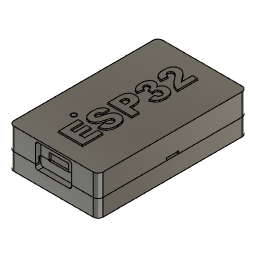
ESP32 BOX YT v12 (Autodesk Fusion 360 design; units mm, degrees)
Autodesk Fusion 360 part; units mm, degrees
(part 1 of 2)
sketch "Sketch1" plane through (0, 0, 0) normal (0, 0, 1) x (1, 0, 0) in component "Board"
  line L0 (13.95, 0) -> (-13.95, 0)
  line L1 (-13.95, 0) -> (-13.95, 54.4)
  line L2 (-13.95, 54.4) -> (13.95, 54.4)
  line L3 (13.95, 54.4) -> (13.95, 0)
  line L4 (13.95, 0) -> (-13.95, 54.4) construction
  line L5 (-13.95, 0) -> (13.95, 54.4) construction
  line L6 (0, 1.75) -> (0, 22.5)
  line L7 (1.75, 0) -> (22.5, 0)
  line L8 (9, 54.4) -> (-9, 54.4)
  line L9 (-9, 54.4) -> (-9, 28.9)
  line L10 (-9, 28.9) -> (9, 28.9)
  line L11 (9, 28.9) -> (9, 54.4)
  line L12 (9, 54.4) -> (-9, 28.9) construction
  line L13 (-9, 54.4) -> (9, 28.9) construction
  line L14 (3.9, 5.7) -> (-3.9, 5.7)
  line L15 (-3.9, 5.7) -> (-3.9, -1)
  line L16 (-3.9, -1) -> (3.9, -1)
  line L17 (3.9, -1) -> (3.9, 5.7)
  line L18 (3.9, 5.7) -> (-3.9, -1) construction
  line L19 (-3.9, 5.7) -> (3.9, -1) construction
  line L20 (-7.6, 13.8) -> (-8.4, 13.8)
  line L21 (-8.4, 13.8) -> (-8.4, 12.2)
  line L22 (-8.4, 12.2) -> (-7.6, 12.2)
  line L23 (-7.6, 12.2) -> (-7.6, 13.8)
  line L24 (-7.6, 13.8) -> (-8.4, 12.2) construction
  line L25 (-8.4, 13.8) -> (-7.6, 12.2) construction
  point P0 (0, 27.2)
  point P1 (0, 41.65)
  point P2 (0, 2.35)
  point P3 (-8, 13)
  dimension "d3" = 27.9
  dimension "d4" = 54.4
  dimension "d5" = 18
  dimension "d6" = 25.5
  dimension "d7" = 7.8
  dimension "d8" = 6.7
  dimension "d9" = 1
  dimension "d10" = 0.8
  dimension "d11" = 1.6
  dimension "d12" = 8
  dimension "d13" = 13
  constraint horizontal L0
  constraint perpendicular L0 L1
  constraint parallel L0 L2
  constraint parallel L1 L3
  constraint coincident L4 P0
  constraint coincident L5 P0
  constraint coincident P0 L6
  constraint collinear L0 L7
  constraint horizontal L8
  constraint perpendicular L8 L9
  constraint parallel L8 L10
  constraint parallel L9 L11
  constraint coincident L12 P1
  constraint coincident L13 P1
  constraint coincident L6 P1
  constraint collinear L2 L8
  constraint horizontal L14
  constraint perpendicular L14 L15
  constraint parallel L14 L16
  constraint parallel L15 L17
  constraint coincident L18 P2
  constraint coincident L19 P2
  constraint coincident L6 P2
  constraint horizontal L20
  constraint perpendicular L20 L21
  constraint parallel L20 L22
  constraint parallel L21 L23
  constraint coincident L24 P3
  constraint coincident L25 P3
  measures "d3" distance of L1.end L2.end
  measures "d4" distance of L0.end L1.end
  measures "d5" distance of L9.end L10.end
  measures "d6" distance of L8.end L9.end
  measures "d7" distance of L15.end L16.end
  measures "d8" distance of L14.end L15.end
  measures "d9" distance of L0 L16
  measures "d10" distance of L21.end L22.end
  measures "d11" distance of L20.end L21.end
  measures "d12" horizontal distance of origin P3
  measures "d13" vertical distance of origin P3
extrude "Extrude1" add sketch "Sketch1" against normal blind 1.6 contours L0 L1 L2 L3 L7 L9 L10 L11 L14 L15 L17 | L0 L7 L14 L15 L17 | L2 L8 L9 L10 L11 | L20 L21 L22 L23 makes body 1 in component "Board"
extrude "Extrude2" add sketch "Sketch1" along normal blind 3.4 contours L2 L8 L9 L10 L11 bodies 1 in component "Board"
extrude "Extrude3" add sketch "Sketch1" along normal blind 0.7 contours L20 L21 L22 L23 bodies 1 in component "Board"
extrude "Extrude4" add sketch "Sketch1" along normal blind 2.7 contours L0 L7 L15 L16 L17 | L0 L7 L14 L15 L17 bodies 1 in component "Board"
extrude "Extrude5" add sketch "Sketch1" against normal blind 0.2 contours L0 L7 L15 L16 L17 bodies 1 in component "Board"
sketch "Sketch1 (2)" plane through (0, 0, 0) normal (0, 0, 1) x (1, 0, 0)
  line L0 (14.25, -0.3) -> (-14.25, -0.3)
  line L1 (-14.25, -0.3) -> (-14.25, 54.7)
  line L2 (-14.25, 54.7) -> (14.25, 54.7)
  line L3 (14.25, 54.7) -> (14.25, -0.3)
  line L4 (14.25, -0.3) -> (-14.25, 54.7) construction
  line L5 (-14.25, -0.3) -> (14.25, 54.7) construction
  line L6 (0, 1.75) -> (0, 22.5)
  line L7 (-17.25, -3.3) -> (-17.25, 57.7)
  line L8 (-17.25, 57.7) -> (17.25, 57.7)
  line L9 (17.25, 57.7) -> (17.25, -3.3)
  line L10 (17.25, -3.3) -> (-17.25, -3.3)
  line L11 (-15.65, -1.7) -> (-15.65, 56.1)
  line L12 (-15.65, 56.1) -> (15.65, 56.1)
  line L13 (15.65, 56.1) -> (15.65, -1.7)
  line L14 (15.65, -1.7) -> (-15.65, -1.7)
  line L15 (-15.85, -1.9) -> (-15.85, 56.3)
  line L16 (-15.85, 56.3) -> (15.85, 56.3)
  line L17 (15.85, 56.3) -> (15.85, -1.9)
  line L18 (15.85, -1.9) -> (-15.85, -1.9)
  line L19 (16.55, 17.4) -> (14.95, 17.4)
  line L20 (14.95, 17.4) -> (14.95, 9.8)
  line L21 (14.95, 9.8) -> (16.55, 9.8)
  line L22 (16.55, 9.8) -> (16.55, 17.4)
  line L23 (16.55, 17.4) -> (14.95, 9.8) construction
  line L24 (14.95, 17.4) -> (16.55, 9.8) construction
  point P0 (0, 27.2)
  point P1 (15.75, 13.6)
  point P2 (15.75, 13.6)
  dimension "d32" = 28.5
  dimension "d33" = 55
  dimension "d34" = 0.3
  dimension "d71" = -1.4
  dimension "d72" = -1.6
  dimension "d100" = 13.6
  dimension "d101" = 15.75
  dimension "d107" = 1.6
  dimension "d108" = 7.6
  constraint horizontal L0
  constraint perpendicular L0 L1
  constraint parallel L0 L2
  constraint parallel L1 L3
  constraint coincident L4 P0
  constraint coincident L5 P0
  constraint coincident P0 L6
  constraint horizontal L19
  constraint perpendicular L19 L20
  constraint parallel L19 L21
  constraint parallel L20 L22
  constraint coincident L23 P2
  constraint coincident L24 P2
  constraint coincident P2 P1
  measures "d32" distance of L1.end L2.end
  measures "d33" distance of L0.end L1.end
  measures "d34" distance of origin L0
  measures "d100" vertical distance of origin P2
  measures "d101" horizontal distance of origin P2
  measures "d107" distance of L20.end L21.end
  measures "d108" distance of L19.end L20.end
extrude "Extrude1'" add sketch "Sketch1 (2)" against normal blind 9 separate body contours L0 L1 L2 L3 | L7 L8 L9 L10 | L11 L12 L13 L14 L15 L16 L17 L18 L19 L21 | L11 L12 L13 L14 L19 L20 L21 | L13 L19 L20 L21 | L13 L17 L19 L21 | L17 L19 L21 L22 makes body 2 in component "Bottom"
extrude "Extrude2'" cut sketch "Sketch1 (2)" against normal blind 8 contours L0 L1 L2 L3 bodies 2 in component "Bottom"
extrude "Extrude1''" add sketch "Sketch1 (2)" along normal blind 7 separate body contours L0 L1 L2 L3 | L7 L8 L9 L10 | L11 L12 L13 L14 L15 L16 L17 L18 L19 L21 | L11 L12 L13 L14 L19 L20 L21 | L13 L19 L20 L21 | L13 L17 L19 L21 | L17 L19 L21 L22 makes body 3 in component "Top"
extrude "Extrude2''" cut sketch "Sketch1 (2)" along normal blind 6 contours L0 L1 L2 L3 bodies 3 in component "Top"
sketch "Sketch1 (3)" plane through (0, 0, -9) normal (0, 0, -1) x (1, 0, 0) in component "Bottom"
  line L0 (17.25, -57.7) -> (17.25, 3.3)
  line L1 (17.25, 3.3) -> (-17.25, 3.3)
  line L2 (-17.25, 3.3) -> (-17.25, -57.7)
  line L3 (-17.25, -57.7) -> (17.25, -57.7)
  line L4 (7.5, -42.2) -> (-7.5, -42.2)
  line L5 (-7.5, -42.2) -> (-7.5, -12.2)
  line L6 (-7.5, -12.2) -> (7.5, -12.2)
  line L7 (7.5, -12.2) -> (7.5, -42.2)
  line L8 (7.5, -42.2) -> (-7.5, -12.2) construction
  line L9 (-7.5, -42.2) -> (7.5, -12.2) construction
  line L10 (0, -1.75) -> (0, -22.5)
  line L11 (16.55, -17.4) -> (14.95, -17.4)
  line L12 (14.95, -17.4) -> (14.95, -9.8)
  line L13 (14.95, -9.8) -> (16.55, -9.8)
  line L14 (16.55, -9.8) -> (16.55, -17.4)
  line L15 (16.55, -17.4) -> (14.95, -9.8) construction
  line L16 (14.95, -17.4) -> (16.55, -9.8) construction
  line L17 (16.55, -19.6) -> (14.95, -19.6)
  line L18 (14.95, -19.6) -> (14.95, -7.6)
  line L19 (14.95, -7.6) -> (16.55, -7.6)
  line L20 (16.55, -7.6) -> (16.55, -19.6)
  line L21 (16.55, -19.6) -> (14.95, -7.6) construction
  line L22 (14.95, -19.6) -> (16.55, -7.6) construction
  point P0 (0, -27.2)
  point P1 (15.75, -13.6)
  point P2 (15.75, -13.6)
  dimension "d56" = 15
  dimension "d57" = 30
  dimension "d58" = 27.2
  dimension "d123" = 1.6
  dimension "d124" = 7.6
  dimension "d125" = 1.6
  dimension "d126" = 12
  dimension "d127" = 15.75
  dimension "d128" = 13.6
  constraint horizontal L4
  constraint perpendicular L4 L5
  constraint parallel L4 L6
  constraint parallel L5 L7
  constraint coincident L8 P0
  constraint coincident L9 P0
  constraint coincident P0 L10
  constraint horizontal L11
  constraint perpendicular L11 L12
  constraint parallel L11 L13
  constraint parallel L12 L14
  constraint coincident L15 P2
  constraint coincident L16 P2
  constraint horizontal L17
  constraint perpendicular L17 L18
  constraint parallel L17 L19
  constraint parallel L18 L20
  constraint coincident L21 P2
  constraint coincident L22 P2
  constraint coincident P2 P1
  measures "d56" distance of L5.end L6.end
  measures "d57" distance of L4.end L5.end
  measures "d58" distance of origin P0
  measures "d123" distance of L12.end L13.end
  measures "d124" distance of L11.end L12.end
  measures "d125" distance of L18.end L19.end
  measures "d126" distance of L17.end L18.end
  measures "d127" horizontal distance of origin P2
  measures "d128" vertical distance of origin P2
extrude "Extrude5'" add sketch "Sketch1 (3)" against normal blind 7.3 contours L4 L5 L6 L7 bodies 2 in component "Bottom"
sketch "Sketch1 (4)" plane through (0, 0, 7) normal (0, 0, 1) x (-1, 0, 0) in component "Top"
  line L0 (-17.25, 3.3) -> (-17.25, -57.7)
  line L1 (-17.25, -57.7) -> (17.25, -57.7)
  line L2 (17.25, -57.7) -> (17.25, 3.3)
  line L3 (17.25, 3.3) -> (-17.25, 3.3)
  line L4 (-5, -34.4) -> (5, -34.4)
  line L5 (5, -34.4) -> (5, -44.4)
  line L6 (5, -44.4) -> (-5, -44.4)
  line L7 (-5, -44.4) -> (-5, -34.4)
  line L8 (-5, -34.4) -> (5, -44.4) construction
  line L9 (5, -34.4) -> (-5, -44.4) construction
  line L10 (-2.5, -0.5) -> (2.5, -0.5)
  line L11 (2.5, -0.5) -> (2.5, -5.5)
  line L12 (2.5, -5.5) -> (-2.5, -5.5)
  line L13 (-2.5, -5.5) -> (-2.5, -0.5)
  line L14 (-2.5, -0.5) -> (2.5, -5.5) construction
  line L15 (2.5, -0.5) -> (-2.5, -5.5) construction
  line L16 (0, -1.75) -> (0, -22.5)
  circle A0 centre (8, -13) radius 1.075
  circle A1 centre (8, -13) radius 3.075
  line L17 (-13.95, 0) -> (-13.95, -54.4) construction
  line L18 (-13.95, -54.4) -> (13.95, -54.4) construction
  line L19 (13.95, -54.4) -> (13.95, 0) construction
  line L20 (13.95, 0) -> (-13.95, 0) construction
  point P0 (0, -39.4)
  point P1 (0, -3)
  point P2 (8, -13)
  dimension "d61" = 10
  dimension "d62" = 10
  dimension "d63" = 5
  dimension "d64" = 5
  dimension "d65" = 3
  dimension "d66" = 39.4
  dimension "d143" = 2.15
  dimension "d144" = 2
  dimension "d162" = 10
  dimension "d163" = 54.4
  dimension "d164" = 27.9
  text T0 "ESP32" font "Arial Black" height 10 align centre middle in box 54.4 x 27.9 at (-13.95, 0) x (0, -1) y (1, 0) spacing 1 kerned
  constraint horizontal L4
  constraint perpendicular L4 L5
  constraint parallel L4 L6
  constraint parallel L5 L7
  constraint coincident L8 P0
  constraint coincident L9 P0
  constraint horizontal L10
  constraint perpendicular L10 L11
  constraint parallel L10 L12
  constraint parallel L11 L13
  constraint coincident L14 P1
  constraint coincident L15 P1
  constraint coincident P0 L16
  constraint coincident P1 L16
  constraint coincident P2 A0.centre
  constraint midpoint origin L20
  constraint vertical L17
  measures "d61" distance of L5.end L6.end
  measures "d62" distance of L4.end L5.end
  measures "d63" distance of L11.end L12.end
  measures "d64" distance of L10.end L11.end
  measures "d65" distance of origin P1
  measures "d66" distance of origin P0
  measures "d143" diameter of A0
extrude "Extrude5''" add sketch "Sketch1 (4)" against normal blind 3.5 contours L4 L5 L6 L7 bodies 3 in component "Top"
extrude "Extrude6" add sketch "Sketch1 (4)" against normal blind 4.2 contours L10 L11 L12 L13 bodies 3 in component "Top"
extrude "Extrude6'" cut sketch "Sketch1 (2)" against normal blind 2 contours L7 L8 L9 L10 | L11 L12 L13 L14 L15 L16 L17 L18 L19 L21 | L13 L17 L19 L21 | L17 L19 L21 L22 bodies 2 in component "Bottom"
extrude "Extrude7" add sketch "Sketch1 (2)" against normal blind 2 contours L7 L8 L9 L10 | L17 L19 L21 L22 bodies 3 in component "Top"
sketch "Sketch2" plane through (0, -3.3, 0) normal (0, -1, 0) x (1, 0, 0)
  line L0 (17.25, -2) -> (17.25, 7)
  line L1 (17.25, 7) -> (-17.25, 7)
  line L2 (-17.25, 7) -> (-17.25, -2)
  line L3 (-3.9, 2.7) -> (3.9, 2.7)
  line L4 (3.9, 2.7) -> (3.9, -0.2)
  line L5 (3.9, -0.2) -> (-3.9, -0.2)
  line L6 (-3.9, -0.2) -> (-3.9, 2.7)
  line L7 (4, -0.3) -> (-4, -0.3)
  line L8 (-4, -0.3) -> (-4, 2.8)
  line L9 (-4, 2.8) -> (4, 2.8)
  line L10 (4, 2.8) -> (4, -0.3)
  line L11 (7.4, -3.7) -> (-7.4, -3.7)
  line L12 (-7.4, -3.7) -> (-7.4, 6.2)
  line L13 (-7.4, 6.2) -> (7.4, 6.2)
  line L14 (7.4, 6.2) -> (7.4, -3.7)
  line L15 (-17.25, -2) -> (17.25, -2)
  dimension "d47" = -3.5
extrude "Extrude3'" cut sketch "Sketch2" against normal blind 3 contours L3 L4 L5 L6 | L7 L8 L9 L10 bodies 2 in component "Bottom"
extrude "Extrude3''" cut sketch "Sketch2" against normal blind 3 contours L3 L4 L5 L6 | L7 L8 L9 L10 bodies 3 in component "Top"
extrude "Extrude4'" cut sketch "Sketch2" against normal blind 2.2 contours L12 L13 L14 L15 | L11 L12 L14 L15 bodies 2 in component "Bottom"
extrude "Extrude4''" cut sketch "Sketch2" against normal blind 2.2 contours L12 L13 L14 L15 | L11 L12 L14 L15 bodies 3 in component "Top"
sketch "Sketch1 (5)" plane through (0, 0, 0) normal (1, 0, 0) x (0, 1, 0) in component "Latch"
  line L0 (0, 1.825) -> (0, 6.175)
  line L1 (0, 6.175) -> (3.5, 6.175)
  line L2 (3.5, 6.175) -> (3.5, -4)
  line L3 (3.5, -4) -> (5, -4.2645)
  line L4 (5, -4.2645) -> (2.5, -8)
  line L5 (2.5, -8) -> (2.5, 1.825)
  line L6 (2.5, 1.825) -> (0, 1.825)
  line L7 (0, 1.75) -> (0, 22.5)
  arc A0 (0, 2.825) -> (0, 5.175) centre (0, 4) ccw
  dimension "d81" = 3.5
  dimension "d82" = 5
  dimension "d85" = 4
  dimension "d86" = 1.175
  dimension "d87" = 4.35
  dimension "d88" = 100
  dimension "d89" = 1
  dimension "d90" = 4
  dimension "d91" = 4
  constraint vertical L0
  constraint perpendicular L0 L1
  constraint perpendicular L1 L2
  constraint parallel L2 L5
  constraint perpendicular L5 L6
  constraint collinear L0 L7
  constraint coincident L0 A0.end
  constraint coincident L7 A0.end
  constraint midpoint L0 A0.centre
  measures "d81" distance of L0.end L1.end
  measures "d82" horizontal distance of origin L3.end
  measures "d85" distance of origin A0.centre
  measures "d86" radius of A0
  measures "d87" distance of L1 L6
  measures "d88" angle of L2 L3
  measures "d89" distance of L2 L5
  measures "d90" vertical distance of origin L2.end
  measures "d91" vertical distance of L2.end L4.end
extrude "Extrude1'''" add sketch "Sketch1 (5)" along normal mid plane 1 separate body contours L0 L1 L2 L3 L4 L5 L6 L7 A0 makes body 4 in component "Latch"
mirror "Mirror1" about plane through (0, 0, 5.175) normal (0, -1, 0) of bodies 4 merged in component "Latch"
ref_plane "WorkPlane1" through (15.75, 13.6, 0) normal (1, 0, 0) x (0, 1, 0)
extrude "Extrude8" cut sketch "Sketch1 (2)" along normal blind 6.475 and the other way blind 2 contours L13 L19 L20 L21 | L13 L17 L19 L21 | L17 L19 L21 L22 bodies 3 in component "Top"
sketch "Sketch2 (2)" plane through (15.75, 13.6, 0) normal (1, 0, 0) x (0, 1, 0) in component "Top"
  circle A0 centre (0, 4) radius 1.175
  line L0 (0, 1.75) -> (0, 22.5)
  line L1 (16.1, -1) -> (11.1, -1)
  line L2 (11.1, -1) -> (11.1, -2)
  line L3 (11.1, -2) -> (16.1, -2)
  line L4 (16.1, -2) -> (16.1, -1)
  line L5 (16.1, -1) -> (11.1, -2) construction
  line L6 (11.1, -1) -> (16.1, -2) construction
  point P0 (13.6, -1.5)
  point P1 (-13.6, 0)
  dimension "d113" = 2.35
  dimension "d114" = 4
  dimension "d137" = 5
  dimension "d138" = 1
  dimension "d139" = 27.2
  dimension "d140" = 2
  constraint coincident A0.centre L0
  constraint horizontal L1
  constraint perpendicular L1 L2
  constraint parallel L1 L3
  constraint parallel L2 L4
  constraint coincident L5 P0
  constraint coincident L6 P0
  measures "d113" diameter of A0
  measures "d114" distance of A0.centre origin
  measures "d137" distance of L2.end L3.end
  measures "d138" distance of L1.end L2.end
  measures "d139" horizontal distance of P0 P1
  measures "d140" distance of L3 P1
extrude "Extrude9" cut sketch "Sketch2 (2)" against normal blind 1.5 contours A0 L0 | A0 L0 bodies 3 in component "Top"
pattern_linear "R-Pattern1" count 1 spacing 0 along (-1, 0, 0) count 2 spacing 27.2 along (0, 1, 0) of "Extrude8", "Extrude9" in component "Top"
extrude "Extrude7'" cut sketch "Sketch1 (3)" against normal blind 9 contours L11 L12 L13 L14 L18 L20 bodies 2 in component "Bottom"
extrude "Extrude8'" cut sketch "Sketch1 (3)" against normal blind 5.2 contours L11 L17 L18 L20 | L13 L18 L19 L20 bodies 2 in component "Bottom"
pattern_linear "R-Pattern1'" count 2 spacing 31.5 along (-1, 0, 0) count 2 spacing 27.2 along (0, 1, 0) of "Extrude7'", "Extrude8'" in component "Bottom"
extrude "Extrude10" cut sketch "Sketch2 (2)" along normal blind 1.5 contours L1 L2 L3 L4 bodies 3 in component "Top"
mirror "Mirror1'" about plane through (0, 0, 0) normal (1, 0, 0) of "Extrude8", "Extrude9", "R-Pattern1", "Extrude10" in component "Top"
extrude "Extrude11" cut sketch "Sketch1 (4)" against normal blind 1 contours A0 bodies 3 in component "Top"
extrude "Extrude12" add sketch "Sketch1 (4)" against normal blind 6 contours A1 bodies 3 in component "Top"
sketch "Sketch1 (6)" plane through (0, 0, 7) normal (0, 0, 1) x (-1, 0, 0) in component "Light Pipe"
  circle A0 centre (8, -13) radius 0.875
  point P0 (8, -13)
  dimension "d149" = 1.75
  constraint coincident P0 A0.centre
  measures "d149" diameter of A0
extrude "Extrude1''''" add sketch "Sketch1 (6)" against normal blind 6 separate body makes body 5 in component "Light Pipe"
fillet "Fillet1" radius 2 4 edges at (17.25, -3.3, 2.5) (17.25, 57.7, 2.5) (-17.25, 57.7, 2.5) (-17.25, -3.3, 2.5) on bodies 3 in component "Top"
fillet "Fillet1'" radius 2 4 edges at (17.25, -3.3, -5.5) (17.25, 57.7, -5.5) (-17.25, 57.7, -5.5) (-17.25, -3.3, -5.5) on bodies 2 in component "Bottom"
fillet "Fillet2" radius 1 2 edges at (-7.4, -2.2, 6.2) (7.4, -2.2, 6.2) on bodies 3 in component "Top"
fillet "Fillet2'" radius 1 2 edges at (-7.4, -2.2, -3.7) (7.4, -2.2, -3.7) on bodies 2 in component "Bottom"
move_face "OffsetFaces1" offset 1 2 faces at (17.25, 28.0333, 4.3333) (-17.25, 26.3667, 4.3333) on bodies 3 in component "Top"
move_face "OffsetFaces1'" offset 1 2 faces at (17.25, 36.7, -4.3333) (-17.25, 17.7, -4.3333) on bodies 2 in component "Bottom"
extrude "Extrude13" cut sketch "Sketch1 (4)" against normal blind 0.5 text T0 bodies 3 in component "Top"
sketch "Sketch1 (7)" plane through (0, 0, 6.5) normal (0, 0, 1) x (-1, 0, 0) in component "Letters"
  line L0 (5, -3.5643) -> (-5, -3.5643)
  line L1 (-5, -3.5643) -> (-5, -11.9954)
  line L2 (-5, -11.9954) -> (-2.7353, -11.9954)
  line L3 (-2.7353, -11.9954) -> (-2.7353, -6.6611)
  line L4 (-2.7353, -6.6611) -> (-0.764, -6.6611)
  line L5 (-0.764, -6.6611) -> (-0.764, -11.4701)
  line L6 (-0.764, -11.4701) -> (1.2756, -11.4701)
  line L7 (1.2756, -11.4701) -> (1.2756, -6.6611)
  line L8 (1.2756, -6.6611) -> (2.8649, -6.6611)
  line L9 (2.8649, -6.6611) -> (2.8649, -11.8453)
  line L10 (2.8649, -11.8453) -> (5, -11.8453)
  line L11 (5, -11.8453) -> (5, -3.5643)
  spline S0 degree 3 poles (-4.1883, -14.2327) (-3.8327, -13.9404) (-3.1037, -13.3409) (-2.17, -13.1954) (-1.6917, -13.1209) knots 0 0 0 0 0.135476 0.277796 0.277796 0.277796 0.277796
  spline S1 degree 3 poles (-5.1705, -17.7662) (-5.1644, -17.0229) (-5.154, -15.7461) (-4.4729, -14.6787) (-4.1883, -14.2327) knots 0 0 0 0 0.217286 0.373233 0.373233 0.373233 0.373233
  spline S2 degree 3 poles (-4.751, -20.1741) (-4.8731, -19.8174) (-5.14, -19.0381) (-5.1598, -18.2134) (-5.1705, -17.7662) knots 0 0 0 0 0.112439 0.245696 0.245696 0.245696 0.245696
  spline S3 degree 3 poles (-3.5198, -21.6611) (-3.7753, -21.4632) (-4.2963, -21.0596) (-4.5975, -20.473) (-4.751, -20.1741) knots 0 0 0 0 0.095714 0.195167 0.195167 0.195167 0.195167
  spline S4 degree 3 poles (-1.7462, -22.1932) (-2.0609, -22.1708) (-2.6918, -22.1259) (-3.2433, -21.8163) (-3.5198, -21.6611) knots 0 0 0 0 0.09338 0.187213 0.187213 0.187213 0.187213
  spline S5 degree 3 poles (-0.266, -21.7941) (-0.4951, -21.9105) (-0.9605, -22.1469) (-1.4817, -22.1776) (-1.7462, -22.1932) knots 0 0 0 0 0.076211 0.15478 0.15478 0.15478 0.15478
  spline S6 degree 3 poles (0.8424, -20.5186) (0.6924, -20.7859) (0.4104, -21.2885) (-0.0503, -21.6329) (-0.266, -21.7941) knots 0 0 0 0 0.090764 0.170661 0.170661 0.170661 0.170661
  spline S7 degree 3 poles (1.7258, -17.6161) (1.5991, -18.2018) (1.3844, -19.1945) (1, -20.1336) (0.8424, -20.5186) knots 0 0 0 0 0.179317 0.303895 0.303895 0.303895 0.303895
  spline S8 degree 3 poles (2.0941, -16.5793) (2.0252, -16.7) (1.8413, -17.022) (1.7702, -17.3876) (1.7258, -17.6161) knots 0 0 0 0 0.041492 0.110653 0.110653 0.110653 0.110653
  spline S9 degree 3 poles (2.5239, -16.3542) (2.4446, -16.3656) (2.2757, -16.39) (2.1571, -16.5137) (2.0941, -16.5793) knots 0 0 0 0 0.023368 0.049766 0.049766 0.049766 0.049766
  spline S10 degree 3 poles (3.0798, -16.627) (3.0009, -16.5474) (2.8468, -16.392) (2.6298, -16.3666) (2.5239, -16.3542) knots 0 0 0 0 0.032559 0.063587 0.063587 0.063587 0.063587
  spline S11 degree 3 poles (3.3083, -17.4387) (3.3039, -17.2769) (3.2958, -16.9857) (3.1462, -16.7373) (3.0798, -16.627) knots 0 0 0 0 0.047582 0.0856 0.0856 0.0856 0.0856
  spline S12 degree 3 poles (3.0014, -18.4653) (3.0907, -18.3218) (3.2856, -18.0088) (3.3004, -17.639) (3.3083, -17.4387) knots 0 0 0 0 0.049883 0.108793 0.108793 0.108793 0.108793
  spline S13 degree 3 poles (2.0191, -18.9531) (2.2226, -18.9107) (2.5942, -18.8334) (2.8746, -18.58) (3.0014, -18.4653) knots 0 0 0 0 0.061034 0.111431 0.111431 0.111431 0.111431
  line L12 (2.0191, -18.9531) -> (2.1896, -21.8658)
  spline S14 degree 3 poles (4.4577, -20.6686) (4.1693, -20.9716) (3.5506, -21.6218) (2.6634, -21.7808) (2.1896, -21.8658) knots 0 0 0 0 0.122331 0.262471 0.262471 0.262471 0.262471
  spline S15 degree 3 poles (5.1705, -17.7457) (5.1574, -18.3209) (5.1338, -19.3515) (4.6649, -20.265) (4.4577, -20.6686) knots 0 0 0 0 0.169849 0.304314 0.304314 0.304314 0.304314
  spline S16 degree 3 poles (4.7783, -15.2866) (4.8923, -15.6383) (5.1509, -16.4361) (5.1635, -17.276) (5.1705, -17.7457) knots 0 0 0 0 0.110321 0.250245 0.250245 0.250245 0.250245
  spline S17 degree 3 poles (3.7005, -13.9428) (3.9196, -14.1171) (4.3797, -14.483) (4.6413, -15.0104) (4.7783, -15.2866) knots 0 0 0 0 0.082926 0.174145 0.174145 0.174145 0.174145
  spline S18 degree 3 poles (2.2442, -13.496) (2.4993, -13.5158) (3.0179, -13.556) (3.4706, -13.8125) (3.7005, -13.9428) knots 0 0 0 0 0.075777 0.154003 0.154003 0.154003 0.154003
  spline S19 degree 3 poles (0.3138, -14.3692) (0.5843, -14.1145) (1.1278, -13.603) (1.871, -13.5318) (2.2442, -13.496) knots 0 0 0 0 0.108188 0.217317 0.217317 0.217317 0.217317
  spline S20 degree 3 poles (-0.9004, -17.2682) (-0.7606, -16.6713) (-0.5177, -15.6338) (0.0659, -14.7461) (0.3138, -14.3692) knots 0 0 0 0 0.182061 0.316451 0.316451 0.316451 0.316451
  spline S21 degree 3 poles (-1.4802, -18.8508) (-1.3727, -18.6652) (-1.088, -18.174) (-0.9724, -17.6157) (-0.9004, -17.2682) knots 0 0 0 0 0.064 0.169461 0.169461 0.169461 0.169461
  spline S22 degree 3 poles (-2.176, -19.1918) (-2.0476, -19.1751) (-1.7782, -19.14) (-1.5826, -18.9502) (-1.4802, -18.8508) knots 0 0 0 0 0.037809 0.079359 0.079359 0.079359 0.079359
  spline S23 degree 3 poles (-2.8956, -18.8337) (-2.7912, -18.9381) (-2.5906, -19.1385) (-2.3103, -19.1745) (-2.176, -19.1918) knots 0 0 0 0 0.042945 0.082429 0.082429 0.082429 0.082429
  spline S24 degree 3 poles (-3.206, -17.8139) (-3.1985, -18.0151) (-3.1847, -18.3839) (-2.986, -18.6931) (-2.8956, -18.8337) knots 0 0 0 0 0.059089 0.108338 0.108338 0.108338 0.108338
  spline S25 degree 3 poles (-2.5989, -16.4497) (-2.7759, -16.6314) (-3.1447, -17.0101) (-3.185, -17.5389) (-3.206, -17.8139) knots 0 0 0 0 0.073722 0.153622 0.153622 0.153622 0.153622
  spline S26 degree 3 poles (-1.5075, -16.0608) (-1.7233, -16.0946) (-2.1127, -16.1554) (-2.4489, -16.3589) (-2.5989, -16.4497) knots 0 0 0 0 0.06474 0.116843 0.116843 0.116843 0.116843
  line L13 (-1.5075, -16.0608) -> (-1.6917, -13.1209)
  line L14 (5, -23.7348) -> (-5, -23.7348)
  line L15 (-5, -23.7348) -> (-5, -26.8385)
  line L16 (-5, -26.8385) -> (-1.2892, -26.8385)
  line L17 (-1.2892, -26.8385) -> (-1.2892, -28.5301)
  spline S27 degree 3 poles (-0.4366, -31.3098) (-0.6845, -30.9379) (-1.2419, -30.1015) (-1.2723, -29.0912) (-1.2892, -28.5301) knots 0 0 0 0 0.131606 0.295937 0.295937 0.295937 0.295937
  spline S28 degree 3 poles (1.9304, -32.2205) (1.4621, -32.1916) (0.574, -32.1367) (-0.1122, -31.5752) (-0.4366, -31.3098) knots 0 0 0 0 0.136799 0.259393 0.259393 0.259393 0.259393
  spline S29 degree 3 poles (4.2019, -31.3849) (3.8929, -31.6283) (3.2295, -32.1508) (2.3827, -32.1962) (1.9304, -32.2205) knots 0 0 0 0 0.115225 0.247344 0.247344 0.247344 0.247344
  spline S30 degree 3 poles (5, -28.8712) (4.9827, -29.3771) (4.9514, -30.2947) (4.4341, -31.0472) (4.2019, -31.3849) knots 0 0 0 0 0.148093 0.268627 0.268627 0.268627 0.268627
  line L18 (5, -28.8712) -> (5, -23.7348)
  line L19 (0.7367, -26.8385) -> (2.9673, -26.8385)
  line L20 (2.9673, -26.8385) -> (2.9673, -27.7184)
  spline S31 degree 3 poles (2.6398, -28.8985) (2.7346, -28.7519) (2.9644, -28.3965) (2.9662, -27.9694) (2.9673, -27.7184) knots 0 0 0 0 0.051432 0.124708 0.124708 0.124708 0.124708
  spline S32 degree 3 poles (1.8417, -29.2123) (1.9921, -29.1998) (2.2897, -29.175) (2.5239, -28.99) (2.6398, -28.8985) knots 0 0 0 0 0.044188 0.087468 0.087468 0.087468 0.087468
  spline S33 degree 3 poles (1.0471, -28.8508) (1.1581, -28.9562) (1.3814, -29.1681) (1.6878, -29.1975) (1.8417, -29.2123) knots 0 0 0 0 0.044579 0.089579 0.089579 0.089579 0.089579
  spline S34 degree 3 poles (0.7367, -27.5956) (0.7385, -27.8559) (0.7415, -28.3021) (0.9572, -28.6893) (1.0471, -28.8508) knots 0 0 0 0 0.076452 0.131111 0.131111 0.131111 0.131111
  line L21 (0.7367, -27.5956) -> (0.7367, -26.8385)
  spline S35 degree 3 poles (3.148, -36.4974) (3.0161, -36.4016) (2.7063, -36.1767) (2.3261, -36.1161) (2.1078, -36.0813) knots 0 0 0 0 0.048282 0.113425 0.113425 0.113425 0.113425
  spline S36 degree 3 poles (3.4447, -37.2955) (3.4344, -37.1416) (3.4146, -36.8455) (3.2345, -36.6104) (3.148, -36.4974) knots 0 0 0 0 0.045123 0.086852 0.086852 0.086852 0.086852
  spline S37 degree 3 poles (3.1719, -38.0458) (3.2514, -37.9421) (3.4205, -37.7215) (3.4363, -37.443) (3.4447, -37.2955) knots 0 0 0 0 0.038322 0.081498 0.081498 0.081498 0.081498
  spline S38 degree 3 poles (2.442, -38.3187) (2.5843, -38.3096) (2.8559, -38.2924) (3.07, -38.1254) (3.1719, -38.0458) knots 0 0 0 0 0.04166 0.079551 0.079551 0.079551 0.079551
  spline S39 degree 3 poles (1.6166, -37.9538) (1.7367, -38.0602) (1.9733, -38.2698) (2.2874, -38.3026) (2.442, -38.3187) knots 0 0 0 0 0.046854 0.092288 0.092288 0.092288 0.092288
  spline S40 degree 3 poles (1.2688, -37.0431) (1.2819, -37.2161) (1.3077, -37.5545) (1.5152, -37.8226) (1.6166, -37.9538) knots 0 0 0 0 0.050801 0.09941 0.09941 0.09941 0.09941
  spline S41 degree 3 poles (1.3029, -36.6816) (1.293, -36.7502) (1.2757, -36.8702) (1.2708, -36.9913) (1.2688, -37.0431) knots 0 0 0 0 0.020792 0.036334 0.036334 0.036334 0.036334
  line L22 (1.3029, -36.6816) -> (-0.6821, -36.5383)
  spline S42 degree 3 poles (-0.5184, -37.4387) (-0.5285, -37.3085) (-0.5521, -37.0031) (-0.6347, -36.7078) (-0.6821, -36.5383) knots 0 0 0 0 0.039096 0.091709 0.091709 0.091709 0.091709
  spline S43 degree 3 poles (-0.9004, -38.4108) (-0.7891, -38.2765) (-0.5559, -37.9953) (-0.5313, -37.6297) (-0.5184, -37.4387) knots 0 0 0 0 0.051012 0.106831 0.106831 0.106831 0.106831
  spline S44 degree 3 poles (-1.9782, -38.7689) (-1.7653, -38.7593) (-1.3706, -38.7414) (-1.0487, -38.5151) (-0.9004, -38.4108) knots 0 0 0 0 0.062379 0.115684 0.115684 0.115684 0.115684
  spline S45 degree 3 poles (-3.0696, -38.3971) (-2.9158, -38.5055) (-2.5895, -38.7354) (-2.1897, -38.7573) (-1.9782, -38.7689) knots 0 0 0 0 0.055294 0.117384 0.117384 0.117384 0.117384
  spline S46 degree 3 poles (-3.4789, -37.466) (-3.462, -37.6445) (-3.4285, -38.0001) (-3.1889, -38.2651) (-3.0696, -38.3971) knots 0 0 0 0 0.052256 0.104169 0.104169 0.104169 0.104169
  spline S47 degree 3 poles (-3.1548, -36.5895) (-3.2493, -36.7149) (-3.4447, -36.9741) (-3.4672, -37.2985) (-3.4789, -37.466) knots 0 0 0 0 0.046068 0.095256 0.095256 0.095256 0.095256
  spline S48 degree 3 poles (-1.9918, -36.0813) (-2.2375, -36.1318) (-2.6632, -36.2192) (-3.0087, -36.4794) (-3.1548, -36.5895) knots 0 0 0 0 0.074035 0.128309 0.128309 0.128309 0.128309
  line L23 (-1.9918, -36.0813) -> (-2.3602, -33.305)
  spline S49 degree 3 poles (-3.912, -34.0861) (-3.6858, -33.9245) (-3.2094, -33.584) (-2.6526, -33.4011) (-2.3602, -33.305) knots 0 0 0 0 0.082898 0.174626 0.174626 0.174626 0.174626
  spline S50 degree 3 poles (-4.8499, -35.3821) (-4.7324, -35.1326) (-4.5011, -34.6414) (-4.1062, -34.2692) (-3.912, -34.0861) knots 0 0 0 0 0.081932 0.161255 0.161255 0.161255 0.161255
  spline S51 degree 3 poles (-5.1705, -37.5342) (-5.1648, -37.1242) (-5.1546, -36.3913) (-4.9431, -35.6907) (-4.8499, -35.3821) knots 0 0 0 0 0.122278 0.218526 0.218526 0.218526 0.218526
  spline S52 degree 3 poles (-4.7374, -39.7921) (-4.8634, -39.4643) (-5.1423, -38.739) (-5.1605, -37.9608) (-5.1705, -37.5342) knots 0 0 0 0 0.104593 0.23142 0.23142 0.23142 0.23142
  spline S53 degree 3 poles (-3.5027, -41.1086) (-3.7553, -40.9379) (-4.2663, -40.5926) (-4.5792, -40.0609) (-4.7374, -39.7921) knots 0 0 0 0 0.090235 0.182525 0.182525 0.182525 0.182525
  spline S54 degree 3 poles (-1.8281, -41.5656) (-2.118, -41.5455) (-2.7065, -41.5047) (-3.2347, -41.2419) (-3.5027, -41.1086) knots 0 0 0 0 0.086282 0.175103 0.175103 0.175103 0.175103
  spline S55 degree 3 poles (-0.631, -41.2894) (-0.8116, -41.3699) (-1.1922, -41.5396) (-1.609, -41.5566) (-1.8281, -41.5656) knots 0 0 0 0 0.05877 0.123854 0.123854 0.123854 0.123854
  spline S56 degree 3 poles (0.1774, -40.5151) (0.0674, -40.6716) (-0.1512, -40.9828) (-0.4717, -41.1876) (-0.631, -41.2894) knots 0 0 0 0 0.056767 0.112893 0.112893 0.112893 0.112893
  spline S57 degree 3 poles (0.5116, -39.6284) (0.4669, -39.8016) (0.3875, -40.1096) (0.2413, -40.3917) (0.1774, -40.5151) knots 0 0 0 0 0.053461 0.095032 0.095032 0.095032 0.095032
  spline S58 degree 3 poles (1.4325, -40.6993) (1.259, -40.559) (0.8875, -40.2584) (0.6423, -39.8474) (0.5116, -39.6284) knots 0 0 0 0 0.066407 0.14223 0.14223 0.14223 0.14223
  spline S59 degree 3 poles (2.6057, -41.054) (2.3954, -41.0396) (1.9771, -41.0109) (1.6133, -40.8028) (1.4325, -40.6993) knots 0 0 0 0 0.062366 0.123997 0.123997 0.123997 0.123997
  spline S60 degree 3 poles (4.4407, -40.1809) (4.1833, -40.4356) (3.673, -40.9406) (2.9595, -41.0164) (2.6057, -41.054) knots 0 0 0 0 0.105226 0.208681 0.208681 0.208681 0.208681
  spline S61 degree 3 poles (5.1705, -37.3501) (5.1621, -37.9272) (5.1474, -38.9358) (4.6524, -39.8078) (4.4407, -40.1809) knots 0 0 0 0 0.169641 0.296487 0.296487 0.296487 0.296487
  spline S62 degree 3 poles (4.502, -34.7136) (4.6965, -35.0811) (5.131, -35.9025) (5.1565, -36.8349) (5.1705, -37.3501) knots 0 0 0 0 0.123135 0.275233 0.275233 0.275233 0.275233
  spline S63 degree 3 poles (2.5784, -33.4551) (2.9683, -33.5839) (3.7225, -33.8329) (4.2481, -34.4268) (4.502, -34.7136) knots 0 0 0 0 0.120727 0.23356 0.23356 0.23356 0.23356
  line L24 (2.5784, -33.4551) -> (2.1078, -36.0813)
  line L25 (-5, -50.8357) -> (-2.7353, -50.8357)
  line L26 (-2.7353, -50.8357) -> (-2.7353, -46.4974)
  spline S64 degree 3 poles (-2.1282, -47.1625) (-2.2165, -47.059) (-2.4113, -46.8304) (-2.6208, -46.6152) (-2.7353, -46.4974) knots 0 0 0 0 0.040795 0.090071 0.090071 0.090071 0.090071
  spline S65 degree 3 poles (-1.3165, -48.2846) (-1.4784, -48.0495) (-1.7403, -47.6691) (-2.021, -47.3025) (-2.1282, -47.1625) knots 0 0 0 0 0.085612 0.138511 0.138511 0.138511 0.138511
  spline S66 degree 3 poles (0.5116, -50.2321) (0.2097, -49.991) (-0.4921, -49.4308) (-1.0173, -48.7006) (-1.3165, -48.2846) knots 0 0 0 0 0.115403 0.268207 0.268207 0.268207 0.268207
  spline S67 degree 3 poles (2.2578, -50.7675) (1.9538, -50.7434) (1.3325, -50.6941) (0.7891, -50.3882) (0.5116, -50.2321) knots 0 0 0 0 0.090356 0.184607 0.184607 0.184607 0.184607
  spline S68 degree 3 poles (3.8097, -50.3003) (3.5709, -50.4366) (3.0895, -50.7112) (2.5365, -50.7487) (2.2578, -50.7675) knots 0 0 0 0 0.081349 0.16395 0.16395 0.16395 0.16395
  spline S69 degree 3 poles (4.8363, -49.0179) (4.7116, -49.274) (4.4658, -49.7789) (4.0263, -50.1281) (3.8097, -50.3003) knots 0 0 0 0 0.084251 0.166139 0.166139 0.166139 0.166139
  spline S70 degree 3 poles (5.1705, -46.7362) (5.1653, -47.1743) (5.1561, -47.9511) (4.9334, -48.694) (4.8363, -49.0179) knots 0 0 0 0 0.130639 0.231601 0.231601 0.231601 0.231601
  spline S71 degree 3 poles (4.8192, -44.5363) (4.9213, -44.8496) (5.1537, -45.563) (5.1645, -46.3146) (5.1705, -46.7362) knots 0 0 0 0 0.098326 0.22389 0.22389 0.22389 0.22389
  spline S72 degree 3 poles (3.8097, -43.3051) (4.0177, -43.4687) (4.4446, -43.8045) (4.6923, -44.2883) (4.8192, -44.5363) knots 0 0 0 0 0.078417 0.160907 0.160907 0.160907 0.160907
  spline S73 degree 3 poles (1.9782, -42.7048) (2.3333, -42.7617) (2.9768, -42.8649) (3.5519, -43.1688) (3.8097, -43.3051) knots 0 0 0 0 0.106995 0.193889 0.193889 0.193889 0.193889
  line L27 (1.9782, -42.7048) -> (1.7531, -45.4879)
  spline S74 degree 3 poles (2.9332, -45.9415) (2.7837, -45.8364) (2.4304, -45.588) (2.0008, -45.5245) (1.7531, -45.4879) knots 0 0 0 0 0.054151 0.127962 0.127962 0.127962 0.127962
  spline S75 degree 3 poles (3.2674, -46.8112) (3.2553, -46.6439) (3.2319, -46.3195) (3.0306, -46.0648) (2.9332, -45.9415) knots 0 0 0 0 0.049062 0.09511 0.09511 0.09511 0.09511
  spline S76 degree 3 poles (2.9434, -47.6604) (3.0379, -47.5386) (3.2317, -47.2888) (3.2553, -46.973) (3.2674, -46.8112) knots 0 0 0 0 0.045202 0.092709 0.092709 0.092709 0.092709
  spline S77 degree 3 poles (2.1623, -47.9981) (2.3095, -47.9837) (2.6058, -47.9546) (2.8304, -47.7589) (2.9434, -47.6604) knots 0 0 0 0 0.04321 0.087001 0.087001 0.087001 0.087001
  spline S78 degree 3 poles (1.2688, -47.657) (1.4165, -47.7563) (1.689, -47.9393) (2.0137, -47.9796) (2.1623, -47.9981) knots 0 0 0 0 0.052523 0.096837 0.096837 0.096837 0.096837
  spline S79 degree 3 poles (-0.1091, -46.095) (0.1444, -46.44) (0.5578, -47.0024) (1.0705, -47.4745) (1.2688, -47.657) knots 0 0 0 0 0.128023 0.208705 0.208705 0.208705 0.208705
  spline S80 degree 3 poles (-2.6774, -43.3699) (-2.2692, -43.7057) (-1.2992, -44.5039) (-0.5456, -45.5113) (-0.1091, -46.095) knots 0 0 0 0 0.158042 0.375637 0.375637 0.375637 0.375637
  spline S81 degree 3 poles (-5, -42.5001) (-4.5922, -42.5738) (-3.7656, -42.723) (-3.0433, -43.1523) (-2.6774, -43.3699) knots 0 0 0 0 0.123237 0.249808 0.249808 0.249808 0.249808
  line L28 (-5, -42.5001) -> (-5, -50.8357)
  line L29 (-2.8353, -11.8954) -> (-2.8353, -6.5611)
  line L30 (-2.8353, -6.5611) -> (-0.664, -6.5611)
  line L31 (-0.664, -6.5611) -> (-0.664, -11.3701)
  line L32 (-0.664, -11.3701) -> (1.1756, -11.3701)
  line L33 (1.1756, -11.3701) -> (1.1756, -6.5611)
  line L34 (1.1756, -6.5611) -> (2.9649, -6.5611)
  line L35 (2.9649, -6.5611) -> (2.9649, -11.7453)
  line L36 (2.9649, -11.7453) -> (4.9, -11.7453)
  line L37 (4.9, -11.7453) -> (4.9, -3.6643)
  line L38 (4.9, -3.6643) -> (-4.9, -3.6643)
  line L39 (-4.9, -3.6643) -> (-4.9, -11.8954)
  line L40 (-4.9, -11.8954) -> (-2.8353, -11.8954)
  spline S82 degree 3 poles (-1.7456, -22.093) (-2.058, -22.0707) (-2.3631, -22.0478) (-2.6419, -21.9644) (-2.9217, -21.8806) (-3.1902, -21.7315) (-3.4644, -21.5775) knots 0.000642 0.000642 0.000642 0.000642 0.09338 0.09338 0.09338 0.186484 0.186484 0.186484 0.186484
  spline S83 degree 3 poles (-3.4644, -21.5775) (-3.7179, -21.3812) (-3.965, -21.1882) (-4.1568, -20.9591) (-4.3562, -20.721) (-4.5064, -20.4315) (-4.6588, -20.1348) knots 0.00073 0.00073 0.00073 0.00073 0.095714 0.095714 0.095714 0.194453 0.194453 0.194453 0.194453
  spline S84 degree 3 poles (-4.6588, -20.1348) (-4.7801, -19.7805) (-4.8993, -19.4304) (-4.9675, -19.0757) (-5.0487, -18.6533) (-5.0598, -18.2121) (-5.0705, -17.7654) knots 0.00072 0.00072 0.00072 0.00072 0.112439 0.112439 0.112439 0.245537 0.245537 0.245537 0.245537
  spline S85 degree 3 poles (-5.0705, -17.7654) (-5.0644, -17.0226) (-5.0564, -16.2908) (-4.8305, -15.64) (-4.6699, -15.1773) (-4.3942, -14.7413) (-4.1125, -14.2999) knots 0.000157 0.000157 0.000157 0.000157 0.217286 0.217286 0.217286 0.371674 0.371674 0.371674 0.371674
  spline S86 degree 3 poles (-4.1125, -14.2999) (-3.7612, -14.011) (-3.4151, -13.7296) (-3.0315, -13.5546) (-2.6547, -13.3827) (-2.2253, -13.306) (-1.7846, -13.2366) knots 0.001556 0.001556 0.001556 0.001556 0.135476 0.135476 0.135476 0.267034 0.267034 0.267034 0.267034
  line L41 (-1.613, -15.9762) -> (-1.7846, -13.2366)
  spline S87 degree 3 poles (-1.613, -15.9762) (-1.8003, -16.0063) (-1.9912, -16.0413) (-2.1747, -16.1126) (-2.3461, -16.1792) (-2.5007, -16.2734) (-2.6507, -16.3641) (-2.6543, -16.3663) (-2.658, -16.3685) (-2.6616, -16.3707) knots 0.008972 0.008972 0.008972 0.008972 0.06474 0.06474 0.06474 0.116843 0.116843 0.116843 0.118111 0.118111 0.118111 0.118111
  spline S88 degree 3 poles (-2.6616, -16.3707) (-2.6646, -16.3738) (-2.6676, -16.3768) (-2.6706, -16.3799) (-2.8475, -16.5616) (-3.0336, -16.7497) (-3.1448, -16.987) (-3.2653, -17.2443) (-3.2847, -17.5313) (-3.3057, -17.8063) (-3.3059, -17.8082) (-3.306, -17.8101) (-3.3061, -17.812) knots -0.001239 -0.001239 -0.001239 -0.001239 0 0 0 0.073722 0.073722 0.073722 0.153622 0.153622 0.153622 0.15417 0.15417 0.15417 0.15417
  spline S89 degree 3 poles (-3.3061, -17.812) (-3.3061, -17.8139) (-3.306, -17.8158) (-3.3059, -17.8177) (-3.2984, -18.0188) (-3.292, -18.2297) (-3.2231, -18.432) (-3.1656, -18.6005) (-3.0701, -18.7472) (-2.9798, -18.8878) (-2.9778, -18.8908) (-2.9759, -18.8938) (-2.9739, -18.8968) knots -0.000556 -0.000556 -0.000556 -0.000556 0 0 0 0.059089 0.059089 0.059089 0.108338 0.108338 0.108338 0.109397 0.109397 0.109397 0.109397
  spline S90 degree 3 poles (-2.9739, -18.8968) (-2.9714, -18.8994) (-2.9689, -18.9019) (-2.9663, -18.9044) (-2.8618, -19.0088) (-2.7509, -19.1227) (-2.6034, -19.1926) (-2.4677, -19.2569) (-2.323, -19.2737) (-2.1887, -19.291) (-2.1845, -19.2915) (-2.1802, -19.2921) (-2.1759, -19.2926) knots -0.001044 -0.001044 -0.001044 -0.001044 0 0 0 0.042945 0.042945 0.042945 0.082429 0.082429 0.082429 0.083686 0.083686 0.083686 0.083686
  spline S91 degree 3 poles (-2.1759, -19.2926) (-2.1716, -19.2921) (-2.1674, -19.2915) (-2.1631, -19.291) (-2.0347, -19.2743) (-1.8962, -19.258) (-1.7655, -19.1972) (-1.6218, -19.1305) (-1.5129, -19.0219) (-1.4106, -18.9225) (-1.4073, -18.9193) (-1.4039, -18.9161) (-1.4006, -18.9129) knots -0.00126 -0.00126 -0.00126 -0.00126 0 0 0 0.037809 0.037809 0.037809 0.079359 0.079359 0.079359 0.080701 0.080701 0.080701 0.080701
  spline S92 degree 3 poles (-1.4006, -18.9129) (-1.3983, -18.9089) (-1.396, -18.9049) (-1.3937, -18.9009) (-1.2862, -18.7154) (-1.1764, -18.5265) (-1.0898, -18.3239) (-0.9473, -17.9905) (-0.8746, -17.6368) (-0.8027, -17.2898) knots -0.001376 -0.001376 -0.001376 -0.001376 0 0 0 0.064 0.064 0.064 0.169333 0.169333 0.169333 0.169333
  spline S93 degree 3 poles (-0.8027, -17.2898) (-0.6631, -16.6933) (-0.5242, -16.1035) (-0.2775, -15.569) (-0.0969, -15.1775) (0.1452, -14.8075) (0.3909, -14.4339) knots 0.000127 0.000127 0.000127 0.000127 0.182061 0.182061 0.182061 0.315284 0.315284 0.315284 0.315284
  spline S94 degree 3 poles (0.3909, -14.4339) (0.6584, -14.1821) (0.9201, -13.94) (1.2164, -13.8054) (1.516, -13.6691) (1.875, -13.6319) (2.2451, -13.5964) knots 0.001141 0.001141 0.001141 0.001141 0.108188 0.108188 0.108188 0.216476 0.216476 0.216476 0.216476
  spline S95 degree 3 poles (2.2451, -13.5964) (2.4972, -13.616) (2.7421, -13.6363) (2.9648, -13.7035) (3.195, -13.7729) (3.4169, -13.897) (3.6444, -14.026) knots 0.000855 0.000855 0.000855 0.000855 0.075777 0.075777 0.075777 0.15323 0.15323 0.15323 0.15323
  spline S96 degree 3 poles (3.6444, -14.026) (3.8613, -14.1985) (4.0721, -14.3678) (4.2356, -14.5658) (4.4158, -14.784) (4.5496, -15.0505) (4.6855, -15.3245) knots 0.000774 0.000774 0.000774 0.000774 0.082926 0.082926 0.082926 0.173419 0.173419 0.173419 0.173419
  spline S97 degree 3 poles (4.6855, -15.3245) (4.7987, -15.6738) (4.91, -16.0191) (4.9741, -16.368) (5.0559, -16.8128) (5.0635, -17.2763) (5.0705, -17.7453) knots 0.000733 0.000733 0.000733 0.000733 0.110321 0.110321 0.110321 0.250057 0.250057 0.250057 0.250057
  spline S98 degree 3 poles (5.0705, -17.7453) (5.0574, -18.3199) (5.0432, -18.886) (4.8961, -19.4077) (4.7807, -19.8168) (4.5802, -20.2109) (4.3753, -20.6101) knots 0.000186 0.000186 0.000186 0.000186 0.169849 0.169849 0.169849 0.30289 0.30289 0.30289 0.30289
  spline S99 degree 3 poles (4.3753, -20.6101) (4.0904, -20.9095) (3.8102, -21.1998) (3.485, -21.384) (3.1376, -21.5807) (2.7176, -21.6686) (2.2829, -21.7474) knots 0.001406 0.001406 0.001406 0.001406 0.122331 0.122331 0.122331 0.251515 0.251515 0.251515 0.251515
  line L42 (2.124, -19.0332) -> (2.2829, -21.7474)
  spline S100 degree 3 poles (2.124, -19.0332) (2.3013, -18.9954) (2.4829, -18.9513) (2.6499, -18.8611) (2.8097, -18.7748) (2.9416, -18.6541) (3.0684, -18.5395) (3.0719, -18.5364) (3.0754, -18.5333) (3.0788, -18.5301) knots 0.008401 0.008401 0.008401 0.008401 0.061034 0.061034 0.061034 0.111431 0.111431 0.111431 0.11281 0.11281 0.11281 0.11281
  spline S101 degree 3 poles (3.0788, -18.5301) (3.0813, -18.5261) (3.0838, -18.5222) (3.0863, -18.5182) (3.1756, -18.3747) (3.2699, -18.2251) (3.3265, -18.0543) (3.3933, -17.8525) (3.4003, -17.643) (3.4082, -17.4427) (3.4083, -17.4416) (3.4083, -17.4405) (3.4084, -17.4394) knots -0.001381 -0.001381 -0.001381 -0.001381 0 0 0 0.049883 0.049883 0.049883 0.108793 0.108793 0.108793 0.109123 0.109123 0.109123 0.109123
  spline S102 degree 3 poles (3.4084, -17.4394) (3.4083, -17.4382) (3.4083, -17.4371) (3.4083, -17.436) (3.4038, -17.2741) (3.4005, -17.1027) (3.3463, -16.9355) (3.303, -16.802) (3.2319, -16.6857) (3.1655, -16.5754) (3.1634, -16.572) (3.1613, -16.5686) (3.1593, -16.5651) knots -0.00033 -0.00033 -0.00033 -0.00033 0 0 0 0.047582 0.047582 0.047582 0.0856 0.0856 0.0856 0.086782 0.086782 0.086782 0.086782
  spline S103 degree 3 poles (3.1593, -16.5651) (3.1564, -16.5623) (3.1536, -16.5594) (3.1508, -16.5566) (3.0719, -16.477) (2.9866, -16.3879) (2.8696, -16.3321) (2.7582, -16.279) (2.6414, -16.2673) (2.5355, -16.2548) (2.5312, -16.2543) (2.5269, -16.2538) (2.5225, -16.2533) knots -0.001164 -0.001164 -0.001164 -0.001164 0 0 0 0.032559 0.032559 0.032559 0.063587 0.063587 0.063587 0.064858 0.064858 0.064858 0.064858
  spline S104 degree 3 poles (2.5225, -16.2533) (2.5182, -16.2539) (2.5139, -16.2546) (2.5096, -16.2552) (2.4303, -16.2667) (2.3407, -16.2778) (2.2532, -16.3206) (2.1542, -16.3689) (2.0849, -16.4444) (2.022, -16.51) (2.0191, -16.513) (2.0163, -16.516) (2.0134, -16.5189) knots -0.001273 -0.001273 -0.001273 -0.001273 0 0 0 0.023368 0.023368 0.023368 0.049766 0.049766 0.049766 0.050963 0.050963 0.050963 0.050963
  spline S105 degree 3 poles (2.0134, -16.5189) (2.0114, -16.5225) (2.0093, -16.5261) (2.0073, -16.5297) (1.9383, -16.6504) (1.8672, -16.7745) (1.8109, -16.909) (1.7172, -17.1328) (1.6722, -17.3678) (1.6278, -17.596) knots -0.001229 -0.001229 -0.001229 -0.001229 0 0 0 0.041492 0.041492 0.041492 0.11055 0.11055 0.11055 0.11055
  spline S106 degree 3 poles (1.6278, -17.596) (1.5012, -18.1814) (1.3751, -18.7634) (1.1916, -19.3235) (1.0647, -19.711) (0.909, -20.0919) (0.7522, -20.475) knots 0.000104 0.000104 0.000104 0.000104 0.179317 0.179317 0.179317 0.303282 0.303282 0.303282 0.303282
  spline S107 degree 3 poles (0.7522, -20.475) (0.6033, -20.7404) (0.4568, -20.9988) (0.2676, -21.2088) (0.1017, -21.3929) (-0.1057, -21.5494) (-0.319, -21.7089) knots 0.000607 0.000607 0.000607 0.000607 0.090764 0.090764 0.090764 0.169809 0.169809 0.169809 0.169809
  spline S108 degree 3 poles (-0.319, -21.7089) (-0.5454, -21.8239) (-0.7665, -21.9348) (-0.9934, -21.997) (-1.228, -22.0613) (-1.4833, -22.0775) (-1.7456, -22.093) knots 0.000852 0.000852 0.000852 0.000852 0.076211 0.076211 0.076211 0.154138 0.154138 0.154138 0.154138
  line L43 (-1.1892, -26.7385) -> (-1.1892, -28.5286)
  spline S109 degree 3 poles (-0.3617, -31.2419) (-0.6067, -30.8743) (-0.8453, -30.5122) (-0.9818, -30.1262) (-1.154, -29.6393) (-1.1724, -29.0891) (-1.1892, -28.5286) knots 0.001469 0.001469 0.001469 0.001469 0.131606 0.131606 0.131606 0.295791 0.295791 0.295791 0.295791
  spline S110 degree 3 poles (1.9308, -32.1203) (1.4645, -32.0915) (1.0092, -32.0609) (0.6196, -31.9003) (0.2732, -31.7576) (-0.0414, -31.504) (-0.3617, -31.2419) knots 0.000561 0.000561 0.000561 0.000561 0.136799 0.136799 0.136799 0.257933 0.257933 0.257933 0.257933
  spline S111 degree 3 poles (4.1281, -31.3157) (3.8232, -31.5558) (3.5241, -31.7879) (3.1978, -31.9187) (2.8203, -32.0701) (2.3811, -32.0961) (1.9308, -32.1203) knots 0.001483 0.001483 0.001483 0.001483 0.115225 0.115225 0.115225 0.246783 0.246783 0.246783 0.246783
  spline S112 degree 3 poles (4.9, -28.8695) (4.8828, -29.3748) (4.864, -29.8696) (4.7065, -30.3046) (4.5797, -30.6547) (4.3573, -30.9824) (4.1281, -31.3157) knots 0.000166 0.000166 0.000166 0.000166 0.148093 0.148093 0.148093 0.267138 0.267138 0.267138 0.267138
  line L44 (4.9, -28.8695) -> (4.9, -23.8348)
  line L45 (4.9, -23.8348) -> (-4.9, -23.8348)
  line L46 (-4.9, -23.8348) -> (-4.9, -26.7385)
  line L47 (-4.9, -26.7385) -> (-1.1892, -26.7385)
  spline S113 degree 3 poles (2.7148, -28.9667) (2.7178, -28.9621) (2.7208, -28.9574) (2.7238, -28.9528) (2.8186, -28.8062) (2.9184, -28.6538) (2.9797, -28.4798) (3.0671, -28.232) (3.0662, -27.9698) (3.0673, -27.7188) (3.0673, -27.7188) (3.0673, -27.7187) (3.0673, -27.7186) knots -0.001627 -0.001627 -0.001627 -0.001627 0 0 0 0.051432 0.051432 0.051432 0.124708 0.124708 0.124708 0.124728 0.124728 0.124728 0.124728
  line L48 (3.0673, -26.7385) -> (3.0673, -27.7186)
  line L49 (0.6367, -26.7385) -> (3.0673, -26.7385)
  line L50 (0.6367, -27.596) -> (0.6367, -26.7385)
  spline S114 degree 3 poles (0.6367, -27.596) (0.6367, -27.5961) (0.6367, -27.5962) (0.6367, -27.5963) (0.6385, -27.8565) (0.6388, -28.1265) (0.7187, -28.3857) (0.7759, -28.571) (0.8698, -28.738) (0.9597, -28.8994) (0.9622, -28.9039) (0.9647, -28.9083) (0.9671, -28.9128) knots -0.000033 -0.000033 -0.000033 -0.000033 0 0 0 0.076452 0.076452 0.076452 0.131111 0.131111 0.131111 0.132617 0.132617 0.132617 0.132617
  spline S115 degree 3 poles (0.9671, -28.9128) (0.9708, -28.9163) (0.9745, -28.9198) (0.9782, -28.9233) (1.0893, -29.0287) (1.2068, -29.1431) (1.3593, -29.2128) (1.5132, -29.2833) (1.6782, -29.297) (1.8322, -29.3118) (1.8352, -29.3121) (1.8381, -29.3124) (1.8411, -29.3127) knots -0.001482 -0.001482 -0.001482 -0.001482 0 0 0 0.044579 0.044579 0.044579 0.089579 0.089579 0.089579 0.090449 0.090449 0.090449 0.090449
  spline S116 degree 3 poles (1.8411, -29.3127) (1.8441, -29.3124) (1.8471, -29.3122) (1.85, -29.3119) (2.0004, -29.2994) (2.1606, -29.2876) (2.3136, -29.2267) (2.4635, -29.1671) (2.5859, -29.0685) (2.7018, -28.977) (2.7061, -28.9736) (2.7105, -28.9701) (2.7148, -28.9667) knots -0.000875 -0.000875 -0.000875 -0.000875 0 0 0 0.044188 0.044188 0.044188 0.087468 0.087468 0.087468 0.089087 0.089087 0.089087 0.089087
  spline S117 degree 3 poles (-4.647, -39.7485) (-4.772, -39.4233) (-4.8944, -39.1027) (-4.9645, -38.7769) (-5.05, -38.3792) (-5.0605, -37.9596) (-5.0705, -37.5338) knots 0.00082 0.00082 0.00082 0.00082 0.104593 0.104593 0.104593 0.231235 0.231235 0.231235 0.231235
  spline S118 degree 3 poles (-5.0705, -37.5338) (-5.0648, -37.1243) (-5.0587, -36.7201) (-4.9918, -36.331) (-4.9395, -36.0267) (-4.8488, -35.7242) (-4.7563, -35.4181) knots 0.000186 0.000186 0.000186 0.000186 0.122278 0.122278 0.122278 0.217794 0.217794 0.217794 0.217794
  spline S119 degree 3 poles (-4.7563, -35.4181) (-4.6399, -35.1709) (-4.5252, -34.9298) (-4.3744, -34.7231) (-4.2283, -34.523) (-4.0409, -34.345) (-3.8483, -34.1635) knots 0.000729 0.000729 0.000729 0.000729 0.081932 0.081932 0.081932 0.160583 0.160583 0.160583 0.160583
  spline S120 degree 3 poles (-3.8483, -34.1635) (-3.6241, -34.0032) (-3.4033, -33.8463) (-3.1695, -33.7256) (-2.9428, -33.6086) (-2.6962, -33.5215) (-2.4434, -33.4378) knots 0.000674 0.000674 0.000674 0.000674 0.082898 0.082898 0.082898 0.162626 0.162626 0.162626 0.162626
  line L51 (-2.1032, -36.0022) -> (-2.4434, -33.4378)
  spline S121 degree 3 poles (-2.1032, -36.0022) (-2.32, -36.0476) (-2.5408, -36.0992) (-2.7463, -36.2005) (-2.9182, -36.2853) (-3.0689, -36.3996) (-3.215, -36.5096) (-3.2188, -36.5124) (-3.2225, -36.5153) (-3.2262, -36.5181) knots 0.009135 0.009135 0.009135 0.009135 0.074035 0.074035 0.074035 0.128309 0.128309 0.128309 0.1297 0.1297 0.1297 0.1297
  spline S122 degree 3 poles (-3.2262, -36.5181) (-3.2291, -36.5218) (-3.2319, -36.5256) (-3.2347, -36.5293) (-3.3292, -36.6547) (-3.4303, -36.7865) (-3.4912, -36.945) (-3.5562, -37.1142) (-3.567, -37.2916) (-3.5786, -37.4591) (-3.5788, -37.4618) (-3.579, -37.4645) (-3.5792, -37.4673) knots -0.001376 -0.001376 -0.001376 -0.001376 0 0 0 0.046068 0.046068 0.046068 0.095256 0.095256 0.095256 0.096056 0.096056 0.096056 0.096056